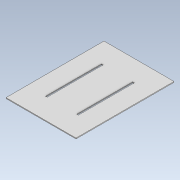
# Autodesk Inventor part: Base
Saved by Autodesk Inventor 2021 (Build 250183000, 183)
## iProperties
Created: 2021-08-28
Part Number: Base
Material: Generic
Document SubType Name: Modeling
Designer: digge
Density: 1 g/cm^3
Appearance: Default
Author: digge
Autodesk Inventor part; units mm, degrees
ref_plane "YZ Plane" through (0, 0, 0) normal (1, 0, 0) x (0, 1, 0)
ref_plane "XZ Plane" through (0, 0, 0) normal (0, 1, 0) x (-1, 0, 0)
ref_plane "XY Plane" through (0, 0, 0) normal (0, 0, 1) x (1, 0, 0)
sketch "Sketch1" plane through (0, 0, 0) normal (0, 1, 0) x (-1, 0, 0)
  line L0 (134.6154, 153.8462) -> (-115.3846, 153.8462)
  line L1 (-115.3846, 153.8462) -> (-115.3846, -196.1538)
  line L2 (-115.3846, -196.1538) -> (134.6154, -196.1538)
  line L3 (134.6154, -196.1538) -> (134.6154, 153.8462)
  line L4 (9.6154, 153.8462) -> (9.6154, -196.1538) construction
  line L5 (134.6154, -21.1538) -> (-115.3846, -21.1538) construction
  line L6 (68.2308, 78.8462) -> (62.2308, 78.8462)
  line L7 (62.2308, 78.8462) -> (62.2308, -121.1538)
  line L8 (62.2308, -121.1538) -> (68.2308, -121.1538)
  line L9 (68.2308, -121.1538) -> (68.2308, 78.8462)
  line L10 (-43, 78.8462) -> (-49, 78.8462)
  line L11 (-49, 78.8462) -> (-49, -121.1538)
  line L12 (-49, -121.1538) -> (-43, -121.1538)
  line L13 (-43, -121.1538) -> (-43, 78.8462)
  point P0 (0, 0)
  dimension "d0" = 250
  dimension "d1" = 350
  dimension "d2" = 6
  dimension "d3" = 6
  dimension "d4" = 200
  constraints: 28 end point, 6 parallel, 4 midpoint, 3 horizontal, 3 perpendicular, 2 collinear, 2 other
  measures "d0" distance of L0.start L0.end
  measures "d1" distance of L2.end L0.start
  measures "d2" distance of L10.start L10.end
  measures "d3" distance of L6.start L6.end
  measures "d4" distance of L8.end L6.start
extrude "Extrusion1" add sketch "Sketch1" along normal blind 3
equation "\"d0\" = BaseDepth"
equation "\"d1\" = BaseLength"
equation "\"d2\" = 2 * Width"
equation "\"d3\" = 2 * Width"
equation "\"d4\" = SlotLength"
equation "\"d5\" = Width"
equation "\"BaseDepth\" = 250"
equation "\"BaseLength\" = 350"
equation "\"Width\" = 3"
equation "\"SlotLength\" = 200"
body "Solid1"
